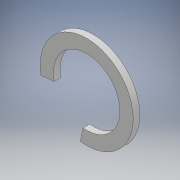
# Autodesk Inventor part: RetainingRingLarge
Saved by Autodesk Inventor 2018 (Build 220112000, 112)
## iProperties
Created: 2017-06-02
Part Number: RetainingRingLarge
Material: Generic
Document SubType Name: Modeling
Designer: Damian
Density: 1 g/cm^3
Appearance: Default
Author: Damian
Autodesk Inventor part; units mm, degrees
ref_plane "YZ Plane" through (0, 0, 0) normal (1, 0, 0) x (0, 1, 0)
ref_plane "XZ Plane" through (0, 0, 0) normal (0, 1, 0) x (-1, 0, 0)
ref_plane "XY Plane" through (0, 0, 0) normal (0, 0, 1) x (1, 0, 0)
sketch "Sketch1" plane through (0, 0, 0) normal (0, 1, 0) x (-1, 0, 0)
  arc A0 (2.1693, 1.9523) -> (0, 0) centre (-0.2733, 2.485) ccw
  arc A1 (3.1653, 1.8326) -> (0.2039, -0.9823) centre (-0.2733, 2.485) ccw
  line L0 (0, 0) -> (0.2039, -0.9823)
  line L1 (2.1693, 1.9523) -> (3.1653, 1.8326)
  dimension "d0" = 2.5
  dimension "d1" = 3.5
  dimension "d2" = 0
  dimension "d3" = 0
  constraints: 4 end point, 4 point on circle, 2 centre point, 1 equal length
  measures "d0" radius of A0
  measures "d1" radius of A1
  measures "d2" distance of A0.centre A1.centre
  measures "d3" distance of A1.centre A0.centre
extrude "Extrusion1" add sketch "Sketch1" along normal blind 0.5
body "Solid1"
